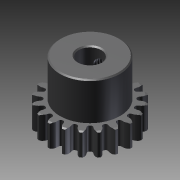
# Autodesk Inventor part: GEAB1.0-20-6-B-6_b
Saved by Autodesk Inventor 2011 SP1 (Build 150282100, 282)
## iProperties
Created: 2016-10-27
Part Number: GEAB1.0-20-6-B-6_b
Catalog Web Link: www.cadenas.de
Description: GEAHB1.0, GEAHBB1.0, GEAHBG1.0, GEAHS1.0, GEAB1.0, GEABB1.0, GEABG1.0, GEAS1.0, GEAKB1.0, GEAKBB1.0, GEAKBG1.0, GEAKS1.0_body-Spur Gears - Pressure Angle 20 Degree Module 1.0
Vendor: MISUMI
Document SubType Name: Modeling
Designer: psAdmin
Manufacturer: MISUMI
Mass: 3.35084 g
Surface Area: 21.074 cm^2
Volume: 3.35084 cm^3
Density: 1 g/cm^3
Category: PARTsolutions
Company: MISUMI
Title: GEAB1.0-20-6-B-6
Author: Cadenas PARTsolutions
Comments: Spur Gears - Pressure Angle 20 Degree Module 1.0
PSOL_IDENT_0: {$CADENAS_DATA\23d-libs\misumi\metric\54_spur_gears\geab10\geab10.prj},460 {VTYP=3D},{NB=GEAB1.0-20-
PSOL_IDENT_1: 6-B-6_b},{LINA=GEAB1.0-20-6-B-6},{NN=GEAHB1.0, GEAHBB1.0, GEAHBG1.0, GEAHS1.0, GEAB1.0, GEABB1.0, GE
PSOL_IDENT_2: ABG1.0, GEAS1.0, GEAKB1.0, GEAKBB1.0, GEAKBG1.0, GEAKS1.0_body},{DATE=13.09.2016 11:19:06},{GEOMDATE=
PSOL_IDENT_3: 13.09.2016 06:08:24},{VERSION=},{LINEID=20},{LINESUBID=-1},{WBVAR=SHS,MAT,ST,NT,B,TS,PS,ALT1,ALT2,TP
PSOL_IDENT_4: C,ALT11,ALT10,BS,ALT4,Z,J,ALT5,Q,R,S,T,ALT9,SRG,ALT6,LFC,LTC,MALT6,ALT7,KFC,KTC,K,ALT3,DIRALT3,QFC,Q
PSOL_IDENT_5: TC,MALT3,ALT8,DIRALT8,ZFC,ZTC,U}  {NB=GEAB1.0-20-6-B-6_b},{LINA=GEAB1.0-20-6-B-6},{KT=DUMMY},{PN=GEA
PSOL_IDENT_6: B1.0-20-6-B-6},{SHS=RHT},{TYPE=GEAB},{MAT=S45C},{MATALG= 'S45C','S45C Equivalent','SUS304','SUS304'
PSOL_IDENT_7: },{ST=},{STALG= '','-','BO','Black Oxide','ENP','Electroless Nickel Plating'},{AC=Set Screw(4137 All
PSOL_IDENT_8: oy Steel Black Oxide)},{MOD=1.0},{NT=20},{NTALG=12,13,14,15,16,17,18,19,20,21,22,23,24,25,26,27,28,2
PSOL_IDENT_9: 9,30,32,34,35,36,38,40,42,44,45,46,48,50,52,54,55,56,58,60,62,64,65,66,68,70,72,75,80,84,85,90,95,96
PSOL_IDENT_10: ,100,110,120},{B=6},{BALG=6,8,10,12},{TS=B},{TSALG='B','B'},{TSPN=-B},{PS=6},{PSALG='6','6','6.35','
PSOL_IDENT_11: 6.35','7','7','8','8','9','9','10','10'},{P=6.00},{DD=20},{D=22},{G=17.5},{H=16},{L=16},{LL1=10},{LL
PSOL_IDENT_12: 2=4},{M=M4},{ML=5.000},{ALT1=},{ALT1ALG='', 'w/o Set Screw', 'KC90','with KC90 (Set Screw)','KC120','
PSOL_IDENT_13: with KC120 (Set Screw)' },{ALT1PN=},{KC=0},{ALT2=},{ALT2ALG= '','w/o TPC (Tapped Hole Dimension)','T
PSOL_IDENT_14: PC','with TPC (Tapped Hole Dimension)' },{TPC=N/A},{TPCALG= 'N/A' },{ALT2PN=},{ALT11=},{ALT11ALG= ''
PSOL_IDENT_15: , 'w/o GBA (Gear bottom adjustment of phase focus)','GBA','with GBA (Gear bottom adjustment of phase
PSOL_IDENT_16: focus)' },{ALT11PN=},{DEG=0},{ALT10=},{ALT10ALG= '','w/o BS (Boss Cut)','BS','with BS (Boss Cut)' }
PSOL_IDENT_17: ,{BS=0.0},{BSALG=0},{BSMIN=7},{BSMAX=10},{ALT10PN=},{LL13D=10},{LL23D=12},{LBS=16},{ALT4=},{ALT4ALG=
PSOL_IDENT_18: '','N/A' },{ALT41=0},{ALT42=0},{ALT4PN=},{Z=0},{ZALG=0},{ZPN=},{ZMINL=8},{ZMAXL=13},{ZMINR=8},{ZMAX
PSOL_IDENT_19: R=12},{J=0.0},{JALG=0},{JPN=},{JMIN=2.0},{JMAX=0.0},{ALT5=},{ALT5ALG= '','N/A' },{ALT5PN=},{Q=0},{QA
PSOL_IDENT_20: LG=0},{QPN=},{QMIN=8},{QMAX=12},{R=0},{RALG=0},{RPN=},{RMIN=8},{RMAX=12.0},{S=0},{SALG=0},{SPN=},{SM
PSOL_IDENT_21: IN=3},{SMAX=10},{T=0},{TALG=0},{TPN=},{TMIN=3},{TMAX=0},{ALT9=},{ALT9ALG= '','Not applicable' },{SRG=
PSOL_IDENT_22: 0.0},{SRGALG=0},{SRGMIN=3.500},{SRGMINALG=3.500},{SRGMAX=0.000},{SRGMAXALG=0.000},{DD2=0.0},{MM=0.00
PSOL_IDENT_23: },{NN=0.00},{DD2ALG=0.000},{MMALG=0.000},{NNALG=0.000},{ALT9PN=},{ALT6=},{ALT6ALG= '','N/A' },{ALT6P
PSOL_IDENT_24: N=},{LFC=0},{LFCALG=0},{LTC=0},{LTCALG=0},{LPCDMIN=14},{LPCDMAX=10},{MALT6=N/A},{MALT6ALG= 'N/A' },{
PSOL_IDENT_25: C=0.0},{ALT7=},{ALT7ALG= '','Not applicable' },{ALT7PN=},{KFC=0},{KFCALG=[0]},{KTC=0},{KTCALG=[0]},{
PSOL_IDENT_26: KPCDMIN1=13},{KPCDMAX1=9},{KPCDMIN2=23},{KPCDMAX2=10},{KPCD=0},{K=0.0},{KALG=[0]},{KALT7L=6},{SCREW=
PSOL_IDENT_27: 4},{SCREWL=5},{ALT3=},{ALT3ALG= '','Not applicable' },{DIRALT3=},{DIRALT3ALG= '','N/A' },{ALT3PN=},{
PSOL_IDENT_28: QFC=0},{QFCALG=[0]},{QTC=0},{QTCALG=[0]},{QPCDMIN1=13},{QPCDMAX1=9},{QPCDMIN2=23},{QPCDMAX2=10},{CIF
PSOL_IDENT_29: MALT3=3},{QPCD=0},{MALT3=N/A},{MALT3ALG= 'N/A' },{MALT3L=0},{MS1=3},{PITCH=0},{BB=0},{TT=0},{ALT8=},
PSOL_IDENT_30: {ALT8ALG= '','Not applicable' },{DIRALT8=},{DIRALT8ALG= '','N/A' },{ALT8PN=},{ZFC=0},{ZFCALG=[0]},{Z
PSOL_IDENT_31: FCMIN=16},{ZFCMAX=7},{ZTC=0},{ZTCALG=[0]},{ZPCDMIN1=16},{ZPCDMIN2=27},{ZPCDMAX1=5},{ZPCDMAX2=7},{ZPC
PSOL_IDENT_32: D=0},{U=0},{UALG=[0]},{UMAX=0},{UMAX1=0},{UMAX2=6},{UMIN=3},{U1=0.0},{U2=0.0},{F=0.0},{PLANE=3},{BL1=
PSOL_IDENT_33: 0},{BL2=15.5},{PCD=0},{SHN=0},{SHDEG1=0},{SHDEG2=0},{PZQRDD2=6},{ALT3LBS=15.5},{D1=4.5},{D2=9},{D3=2
PSOL_IDENT_34: 0},{D4=0.1},{D5=3.333333},{D6=3.076923},{D7=0.85},{D8=0.5},{D9=0.814203},{S1=15},{S2=0.5},{KR=18.16}
NN: 0.00
NT: 20
NB: GEAB1.0-20-6-B-6_b
NBSYN: $PN._b
LINA: GEAB1.0-20-6-B-6
PN: GEAB1.0-20-6-B-6
SHS: Round Hole+Tap
MAT: S45C Equivalent
ST: -
AC: Set Screw(4137 Alloy Steel Black Oxide)
MOD: 1.0
B: 6
TS: B
PS: 6
DD: 20
D: 22
G: 17.5
H: 16
L: 16
LL1: 10
LL2: 4
M: M4
ALT1: w/o Set Screw
ALT2: w/o TPC (Tapped Hole Dimension)
TPC: N/A
ALT11: w/o GBA (Gear bottom adjustment of phase focus)
ALT10: w/o BS (Boss Cut)
BS: 0.0
ALT4: N/A
Z: 0
J: 0.0
ALT5: N/A
Q: 0
R: 0
S: 0
T: 0
ALT9: Not applicable
SRG: 0.0
DD2: 0.0
MM: 0.00
ALT6: N/A
LFC: 0
LTC: 0
MALT6: N/A
C: 0.0
ALT7: Not applicable
KFC: 0
KTC: 0
K: 0.0
ALT3: Not applicable
DIRALT3: N/A
QFC: 0
QTC: 0
MALT3: N/A
ALT8: Not applicable
DIRALT8: N/A
ZFC: 0
ZTC: 0
U: 0
U1: 0.0
U2: 0.0
F: 0.0
SUPPLIER: MISUMI
ARTICLENO: GEAB1.0-20-6-B-6_b
BOMINFO: GEAB1.0-20-6-B-6
CREATOR: CADENAS GmbH
Autodesk Inventor part; units mm, degrees
sketch "Sketch_2" plane through (0, 0, 0) normal (1, 0, 0) x (0, 1, 0)
  line L0 (0, -500) -> (0, 500)
  line L1 (0, 16) -> (7.7, 16)
  line L2 (7.7, 16) -> (8, 15.7)
  line L3 (8, 15.7) -> (8, 6)
  line L4 (8, 6) -> (10.5, 6)
  line L5 (10.5, 6) -> (16, 4.5263)
  line L6 (16, 4.5263) -> (16, 1.4737)
  line L7 (16, 1.4737) -> (10.5, 0)
  line L8 (10.5, 0) -> (0, 0)
  line L9 (0, 0) -> (0, 16)
  constraints: 20 end point
revolve "Revolution1" add sketch "Sketch_2" angle 360 about axis through (0, 0, -500) along (0, 0, -1)
sketch "Sketch_3" plane through (0, 0, 0) normal (0, 0, 1) x (1, 0, 0)
  circle A0 centre (0, 0) radius 44
  arc A1 (-10.9972, 0.248) -> (-10.9972, -0.248) centre (0, 0) ccw
  arc A2 (-10.9972, -0.248) -> (-10.9535, -0.3284) centre (-10.8972, -0.2457) ccw
  arc A3 (-10.9535, -0.3284) -> (-9.9692, -0.7846) centre (-9.0784, 2.4275) ccw
  arc A4 (-9.9692, -0.7846) -> (-9.7201, -0.8136) centre (-9.7516, 0) ccw
  arc A5 (-9.0629, -0.8592) -> (-9.7201, -0.8136) centre (-9.6034, -3.8883) ccw
  arc A6 (-8.6561, -1.2784) -> (-9.0629, -0.8592) centre (-9.1507, -1.3514) ccw
  arc A7 (-8.6561, -1.2784) -> (-8.6275, -1.4591) centre (0, 0) ccw
  arc A8 (-8.8849, -1.9834) -> (-8.6275, -1.4591) centre (-9.1205, -1.5424) ccw
  arc A9 (-9.4958, -2.2299) -> (-8.8849, -1.9834) centre (-10.3349, 0.7304) ccw
  arc A10 (-9.4958, -2.2299) -> (-9.7237, -2.3345) centre (-9.2743, -3.0134) ccw
  arc A11 (-9.7237, -2.3345) -> (-10.5189, -3.0725) centre (-7.8839, -5.1141) ccw
  arc A12 (-10.5189, -3.0725) -> (-10.5356, -3.1625) centre (-10.4398, -3.1337) ccw
  arc A13 (-10.5356, -3.1625) -> (-10.3823, -3.6342) centre (0, 0) ccw
  arc A14 (-10.3823, -3.6342) -> (-10.3159, -3.6971) centre (-10.2879, -3.6011) ccw
  arc A15 (-10.3159, -3.6971) -> (-9.2388, -3.8268) centre (-9.3842, -0.4967) ccw
  arc A16 (-9.2388, -3.8268) -> (-8.993, -3.7775) centre (-9.2743, -3.0134) ccw
  arc A17 (-8.3538, -3.6178) -> (-8.993, -3.7775) centre (-7.9318, -6.6656) ccw
  arc A18 (-7.8374, -3.8907) -> (-8.3538, -3.6178) centre (-8.2853, -4.113) ccw
  arc A19 (-7.8374, -3.8907) -> (-7.7544, -4.0537) centre (0, 0) ccw
  arc A20 (-7.8371, -4.6319) -> (-7.7544, -4.0537) centre (-8.1975, -4.2853) ccw
  arc A21 (-8.342, -5.0551) -> (-7.8371, -4.6319) centre (-10.0548, -2.499) ccw
  arc A22 (-8.342, -5.0551) -> (-8.5264, -5.225) centre (-7.8892, -5.7318) ccw
  arc A23 (-8.5264, -5.225) -> (-9.0546, -6.1726) centre (-5.9177, -7.3) ccw
  arc A24 (-9.0546, -6.1726) -> (-9.0427, -6.2634) centre (-8.9605, -6.2064) ccw
  arc A25 (-9.0427, -6.2634) -> (-8.7512, -6.6646) centre (0, 0) ccw
  arc A26 (-8.7512, -6.6646) -> (-8.6685, -6.704) centre (-8.6716, -6.604) ccw
  arc A27 (-8.6685, -6.704) -> (-7.6041, -6.4945) centre (-8.7714, -3.3722) ccw
  arc A28 (-7.6041, -6.4945) -> (-7.3855, -6.3716) centre (-7.8892, -5.7318) ccw
  arc A29 (-6.827, -6.0222) -> (-7.3855, -6.3716) centre (-5.4838, -8.7904) ccw
  arc A30 (-6.2515, -6.1222) -> (-6.827, -6.0222) centre (-6.6088, -6.472) ccw
  arc A31 (-6.2515, -6.1222) -> (-6.1222, -6.2515) centre (0, 0) ccw
  arc A32 (-6.0222, -6.827) -> (-6.1222, -6.2515) centre (-6.472, -6.6088) ccw
  arc A33 (-6.3716, -7.3855) -> (-6.0222, -6.827) centre (-8.7904, -5.4838) ccw
  arc A34 (-6.3716, -7.3855) -> (-6.4945, -7.6041) centre (-5.7318, -7.8892) ccw
  arc A35 (-6.4945, -7.6041) -> (-6.704, -8.6685) centre (-3.3722, -8.7714) ccw
  arc A36 (-6.704, -8.6685) -> (-6.6646, -8.7512) centre (-6.604, -8.6716) ccw
  arc A37 (-6.6646, -8.7512) -> (-6.2634, -9.0427) centre (0, 0) ccw
  arc A38 (-6.2634, -9.0427) -> (-6.1726, -9.0546) centre (-6.2064, -8.9605) ccw
  arc A39 (-6.1726, -9.0546) -> (-5.225, -8.5264) centre (-7.3, -5.9177) ccw
  arc A40 (-5.225, -8.5264) -> (-5.0551, -8.342) centre (-5.7318, -7.8892) ccw
  arc A41 (-4.6319, -7.8371) -> (-5.0551, -8.342) centre (-2.499, -10.0548) ccw
  arc A42 (-4.0537, -7.7544) -> (-4.6319, -7.8371) centre (-4.2853, -8.1975) ccw
  arc A43 (-4.0537, -7.7544) -> (-3.8907, -7.8374) centre (0, 0) ccw
  arc A44 (-3.6178, -8.3538) -> (-3.8907, -7.8374) centre (-4.113, -8.2853) ccw
  arc A45 (-3.7775, -8.993) -> (-3.6178, -8.3538) centre (-6.6656, -7.9318) ccw
  arc A46 (-3.7775, -8.993) -> (-3.8268, -9.2388) centre (-3.0134, -9.2743) ccw
  arc A47 (-3.8268, -9.2388) -> (-3.6971, -10.3159) centre (-0.4967, -9.3842) ccw
  arc A48 (-3.6971, -10.3159) -> (-3.6342, -10.3823) centre (-3.6011, -10.2879) ccw
  arc A49 (-3.6342, -10.3823) -> (-3.1625, -10.5356) centre (0, 0) ccw
  arc A50 (-3.1625, -10.5356) -> (-3.0725, -10.5189) centre (-3.1337, -10.4398) ccw
  arc A51 (-3.0725, -10.5189) -> (-2.3345, -9.7237) centre (-5.1141, -7.8839) ccw
  arc A52 (-2.3345, -9.7237) -> (-2.2299, -9.4958) centre (-3.0134, -9.2743) ccw
  arc A53 (-1.9834, -8.8849) -> (-2.2299, -9.4958) centre (0.7304, -10.3349) ccw
  arc A54 (-1.4591, -8.6275) -> (-1.9834, -8.8849) centre (-1.5424, -9.1205) ccw
  arc A55 (-1.4591, -8.6275) -> (-1.2784, -8.6561) centre (0, 0) ccw
  arc A56 (-0.8592, -9.0629) -> (-1.2784, -8.6561) centre (-1.3514, -9.1507) ccw
  arc A57 (-0.8136, -9.7201) -> (-0.8592, -9.0629) centre (-3.8883, -9.6034) ccw
  arc A58 (-0.8136, -9.7201) -> (-0.7846, -9.9692) centre (0, -9.7516) ccw
  arc A59 (-0.7846, -9.9692) -> (-0.3284, -10.9535) centre (2.4275, -9.0784) ccw
  arc A60 (-0.3284, -10.9535) -> (-0.248, -10.9972) centre (-0.2457, -10.8972) ccw
  arc A61 (-0.248, -10.9972) -> (0.248, -10.9972) centre (0, 0) ccw
  arc A62 (0.248, -10.9972) -> (0.3284, -10.9535) centre (0.2457, -10.8972) ccw
  arc A63 (0.3284, -10.9535) -> (0.7846, -9.9692) centre (-2.4275, -9.0784) ccw
  arc A64 (0.7846, -9.9692) -> (0.8136, -9.7201) centre (0, -9.7516) ccw
  arc A65 (0.8592, -9.0629) -> (0.8136, -9.7201) centre (3.8883, -9.6034) ccw
  arc A66 (1.2784, -8.6561) -> (0.8592, -9.0629) centre (1.3514, -9.1507) ccw
  arc A67 (1.2784, -8.6561) -> (1.4591, -8.6275) centre (0, 0) ccw
  arc A68 (1.9834, -8.8849) -> (1.4591, -8.6275) centre (1.5424, -9.1205) ccw
  arc A69 (2.2299, -9.4958) -> (1.9834, -8.8849) centre (-0.7304, -10.3349) ccw
  arc A70 (2.2299, -9.4958) -> (2.3345, -9.7237) centre (3.0134, -9.2743) ccw
  arc A71 (2.3345, -9.7237) -> (3.0725, -10.5189) centre (5.1141, -7.8839) ccw
  arc A72 (3.0725, -10.5189) -> (3.1625, -10.5356) centre (3.1337, -10.4398) ccw
  arc A73 (3.1625, -10.5356) -> (3.6342, -10.3823) centre (0, 0) ccw
  arc A74 (3.6342, -10.3823) -> (3.6971, -10.3159) centre (3.6011, -10.2879) ccw
  arc A75 (3.6971, -10.3159) -> (3.8268, -9.2388) centre (0.4967, -9.3842) ccw
  arc A76 (3.8268, -9.2388) -> (3.7775, -8.993) centre (3.0134, -9.2743) ccw
  arc A77 (3.6178, -8.3538) -> (3.7775, -8.993) centre (6.6656, -7.9318) ccw
  arc A78 (3.8907, -7.8374) -> (3.6178, -8.3538) centre (4.113, -8.2853) ccw
  arc A79 (3.8907, -7.8374) -> (4.0537, -7.7544) centre (0, 0) ccw
  arc A80 (4.6319, -7.8371) -> (4.0537, -7.7544) centre (4.2853, -8.1975) ccw
  arc A81 (5.0551, -8.342) -> (4.6319, -7.8371) centre (2.499, -10.0548) ccw
  arc A82 (5.0551, -8.342) -> (5.225, -8.5264) centre (5.7318, -7.8892) ccw
  arc A83 (5.225, -8.5264) -> (6.1726, -9.0546) centre (7.3, -5.9177) ccw
  arc A84 (6.1726, -9.0546) -> (6.2634, -9.0427) centre (6.2064, -8.9605) ccw
  arc A85 (6.2634, -9.0427) -> (6.6646, -8.7512) centre (0, 0) ccw
  arc A86 (6.6646, -8.7512) -> (6.704, -8.6685) centre (6.604, -8.6716) ccw
  arc A87 (6.704, -8.6685) -> (6.4945, -7.6041) centre (3.3722, -8.7714) ccw
  arc A88 (6.4945, -7.6041) -> (6.3716, -7.3855) centre (5.7318, -7.8892) ccw
  arc A89 (6.0222, -6.827) -> (6.3716, -7.3855) centre (8.7904, -5.4838) ccw
  arc A90 (6.1222, -6.2515) -> (6.0222, -6.827) centre (6.472, -6.6088) ccw
  arc A91 (6.1222, -6.2515) -> (6.2515, -6.1222) centre (0, 0) ccw
  arc A92 (6.827, -6.0222) -> (6.2515, -6.1222) centre (6.6088, -6.472) ccw
  arc A93 (7.3855, -6.3716) -> (6.827, -6.0222) centre (5.4838, -8.7904) ccw
  arc A94 (7.3855, -6.3716) -> (7.6041, -6.4945) centre (7.8892, -5.7318) ccw
  arc A95 (7.6041, -6.4945) -> (8.6685, -6.704) centre (8.7714, -3.3722) ccw
  arc A96 (8.6685, -6.704) -> (8.7512, -6.6646) centre (8.6716, -6.604) ccw
  arc A97 (8.7512, -6.6646) -> (9.0427, -6.2634) centre (0, 0) ccw
  arc A98 (9.0427, -6.2634) -> (9.0546, -6.1726) centre (8.9605, -6.2064) ccw
  arc A99 (9.0546, -6.1726) -> (8.5264, -5.225) centre (5.9177, -7.3) ccw
  arc A100 (8.5264, -5.225) -> (8.342, -5.0551) centre (7.8892, -5.7318) ccw
  arc A101 (7.8371, -4.6319) -> (8.342, -5.0551) centre (10.0548, -2.499) ccw
  arc A102 (7.7544, -4.0537) -> (7.8371, -4.6319) centre (8.1975, -4.2853) ccw
  arc A103 (7.7544, -4.0537) -> (7.8374, -3.8907) centre (0, 0) ccw
  arc A104 (8.3538, -3.6178) -> (7.8374, -3.8907) centre (8.2853, -4.113) ccw
  arc A105 (8.993, -3.7775) -> (8.3538, -3.6178) centre (7.9318, -6.6656) ccw
  arc A106 (8.993, -3.7775) -> (9.2388, -3.8268) centre (9.2743, -3.0134) ccw
  arc A107 (9.2388, -3.8268) -> (10.3159, -3.6971) centre (9.3842, -0.4967) ccw
  arc A108 (10.3159, -3.6971) -> (10.3823, -3.6342) centre (10.2879, -3.6011) ccw
  arc A109 (10.3823, -3.6342) -> (10.5356, -3.1625) centre (0, 0) ccw
  arc A110 (10.5356, -3.1625) -> (10.5189, -3.0725) centre (10.4398, -3.1337) ccw
  arc A111 (10.5189, -3.0725) -> (9.7237, -2.3345) centre (7.8839, -5.1141) ccw
  arc A112 (9.7237, -2.3345) -> (9.4958, -2.2299) centre (9.2743, -3.0134) ccw
  arc A113 (8.8849, -1.9834) -> (9.4958, -2.2299) centre (10.3349, 0.7304) ccw
  arc A114 (8.6275, -1.4591) -> (8.8849, -1.9834) centre (9.1205, -1.5424) ccw
  arc A115 (8.6275, -1.4591) -> (8.6561, -1.2784) centre (0, 0) ccw
  arc A116 (9.0629, -0.8592) -> (8.6561, -1.2784) centre (9.1507, -1.3514) ccw
  arc A117 (9.7201, -0.8136) -> (9.0629, -0.8592) centre (9.6034, -3.8883) ccw
  arc A118 (9.7201, -0.8136) -> (9.9692, -0.7846) centre (9.7516, 0) ccw
  arc A119 (9.9692, -0.7846) -> (10.9535, -0.3284) centre (9.0784, 2.4275) ccw
  arc A120 (10.9535, -0.3284) -> (10.9972, -0.248) centre (10.8972, -0.2457) ccw
  arc A121 (10.9972, -0.248) -> (10.9972, 0.248) centre (0, 0) ccw
  arc A122 (10.9972, 0.248) -> (10.9535, 0.3284) centre (10.8972, 0.2457) ccw
  arc A123 (10.9535, 0.3284) -> (9.9692, 0.7846) centre (9.0784, -2.4275) ccw
  arc A124 (9.9692, 0.7846) -> (9.7201, 0.8136) centre (9.7516, 0) ccw
  arc A125 (9.0629, 0.8592) -> (9.7201, 0.8136) centre (9.6034, 3.8883) ccw
  arc A126 (8.6561, 1.2784) -> (9.0629, 0.8592) centre (9.1507, 1.3514) ccw
  arc A127 (8.6561, 1.2784) -> (8.6275, 1.4591) centre (0, 0) ccw
  arc A128 (8.8849, 1.9834) -> (8.6275, 1.4591) centre (9.1205, 1.5424) ccw
  arc A129 (9.4958, 2.2299) -> (8.8849, 1.9834) centre (10.3349, -0.7304) ccw
  arc A130 (9.4958, 2.2299) -> (9.7237, 2.3345) centre (9.2743, 3.0134) ccw
  arc A131 (9.7237, 2.3345) -> (10.5189, 3.0725) centre (7.8839, 5.1141) ccw
  arc A132 (10.5189, 3.0725) -> (10.5356, 3.1625) centre (10.4398, 3.1337) ccw
  arc A133 (10.5356, 3.1625) -> (10.3823, 3.6342) centre (0, 0) ccw
  arc A134 (10.3823, 3.6342) -> (10.3159, 3.6971) centre (10.2879, 3.6011) ccw
  arc A135 (10.3159, 3.6971) -> (9.2388, 3.8268) centre (9.3842, 0.4967) ccw
  arc A136 (9.2388, 3.8268) -> (8.993, 3.7775) centre (9.2743, 3.0134) ccw
  arc A137 (8.3538, 3.6178) -> (8.993, 3.7775) centre (7.9318, 6.6656) ccw
  arc A138 (7.8374, 3.8907) -> (8.3538, 3.6178) centre (8.2853, 4.113) ccw
  arc A139 (7.8374, 3.8907) -> (7.7544, 4.0537) centre (0, 0) ccw
  arc A140 (7.8371, 4.6319) -> (7.7544, 4.0537) centre (8.1975, 4.2853) ccw
  arc A141 (8.342, 5.0551) -> (7.8371, 4.6319) centre (10.0548, 2.499) ccw
  arc A142 (8.342, 5.0551) -> (8.5264, 5.225) centre (7.8892, 5.7318) ccw
  arc A143 (8.5264, 5.225) -> (9.0546, 6.1726) centre (5.9177, 7.3) ccw
  arc A144 (9.0546, 6.1726) -> (9.0427, 6.2634) centre (8.9605, 6.2064) ccw
  arc A145 (9.0427, 6.2634) -> (8.7512, 6.6646) centre (0, 0) ccw
  arc A146 (8.7512, 6.6646) -> (8.6685, 6.704) centre (8.6716, 6.604) ccw
  arc A147 (8.6685, 6.704) -> (7.6041, 6.4945) centre (8.7714, 3.3722) ccw
  arc A148 (7.6041, 6.4945) -> (7.3855, 6.3716) centre (7.8892, 5.7318) ccw
  arc A149 (6.827, 6.0222) -> (7.3855, 6.3716) centre (5.4838, 8.7904) ccw
  arc A150 (6.2515, 6.1222) -> (6.827, 6.0222) centre (6.6088, 6.472) ccw
  arc A151 (6.2515, 6.1222) -> (6.1222, 6.2515) centre (0, 0) ccw
  arc A152 (6.0222, 6.827) -> (6.1222, 6.2515) centre (6.472, 6.6088) ccw
  arc A153 (6.3716, 7.3855) -> (6.0222, 6.827) centre (8.7904, 5.4838) ccw
  arc A154 (6.3716, 7.3855) -> (6.4945, 7.6041) centre (5.7318, 7.8892) ccw
  arc A155 (6.4945, 7.6041) -> (6.704, 8.6685) centre (3.3722, 8.7714) ccw
  arc A156 (6.704, 8.6685) -> (6.6646, 8.7512) centre (6.604, 8.6716) ccw
  arc A157 (6.6646, 8.7512) -> (6.2634, 9.0427) centre (0, 0) ccw
  arc A158 (6.2634, 9.0427) -> (6.1726, 9.0546) centre (6.2064, 8.9605) ccw
  arc A159 (6.1726, 9.0546) -> (5.225, 8.5264) centre (7.3, 5.9177) ccw
  arc A160 (5.225, 8.5264) -> (5.0551, 8.342) centre (5.7318, 7.8892) ccw
  arc A161 (4.6319, 7.8371) -> (5.0551, 8.342) centre (2.499, 10.0548) ccw
  arc A162 (4.0537, 7.7544) -> (4.6319, 7.8371) centre (4.2853, 8.1975) ccw
  arc A163 (4.0537, 7.7544) -> (3.8907, 7.8374) centre (0, 0) ccw
  arc A164 (3.6178, 8.3538) -> (3.8907, 7.8374) centre (4.113, 8.2853) ccw
  arc A165 (3.7775, 8.993) -> (3.6178, 8.3538) centre (6.6656, 7.9318) ccw
  arc A166 (3.7775, 8.993) -> (3.8268, 9.2388) centre (3.0134, 9.2743) ccw
  arc A167 (3.8268, 9.2388) -> (3.6971, 10.3159) centre (0.4967, 9.3842) ccw
  arc A168 (3.6971, 10.3159) -> (3.6342, 10.3823) centre (3.6011, 10.2879) ccw
  arc A169 (3.6342, 10.3823) -> (3.1625, 10.5356) centre (0, 0) ccw
  arc A170 (3.1625, 10.5356) -> (3.0725, 10.5189) centre (3.1337, 10.4398) ccw
  arc A171 (3.0725, 10.5189) -> (2.3345, 9.7237) centre (5.1141, 7.8839) ccw
  arc A172 (2.3345, 9.7237) -> (2.2299, 9.4958) centre (3.0134, 9.2743) ccw
  arc A173 (1.9834, 8.8849) -> (2.2299, 9.4958) centre (-0.7304, 10.3349) ccw
  arc A174 (1.4591, 8.6275) -> (1.9834, 8.8849) centre (1.5424, 9.1205) ccw
  arc A175 (1.4591, 8.6275) -> (1.2784, 8.6561) centre (0, 0) ccw
  arc A176 (0.8592, 9.0629) -> (1.2784, 8.6561) centre (1.3514, 9.1507) ccw
  arc A177 (0.8136, 9.7201) -> (0.8592, 9.0629) centre (3.8883, 9.6034) ccw
  arc A178 (0.8136, 9.7201) -> (0.7846, 9.9692) centre (0, 9.7516) ccw
  arc A179 (0.7846, 9.9692) -> (0.3284, 10.9535) centre (-2.4275, 9.0784) ccw
  arc A180 (0.3284, 10.9535) -> (0.248, 10.9972) centre (0.2457, 10.8972) ccw
  arc A181 (0.248, 10.9972) -> (-0.248, 10.9972) centre (0, 0) ccw
  arc A182 (-0.248, 10.9972) -> (-0.3284, 10.9535) centre (-0.2457, 10.8972) ccw
  arc A183 (-0.3284, 10.9535) -> (-0.7846, 9.9692) centre (2.4275, 9.0784) ccw
  arc A184 (-0.7846, 9.9692) -> (-0.8136, 9.7201) centre (0, 9.7516) ccw
  arc A185 (-0.8592, 9.0629) -> (-0.8136, 9.7201) centre (-3.8883, 9.6034) ccw
  arc A186 (-1.2784, 8.6561) -> (-0.8592, 9.0629) centre (-1.3514, 9.1507) ccw
  arc A187 (-1.2784, 8.6561) -> (-1.4591, 8.6275) centre (0, 0) ccw
  arc A188 (-1.9834, 8.8849) -> (-1.4591, 8.6275) centre (-1.5424, 9.1205) ccw
  arc A189 (-2.2299, 9.4958) -> (-1.9834, 8.8849) centre (0.7304, 10.3349) ccw
  arc A190 (-2.2299, 9.4958) -> (-2.3345, 9.7237) centre (-3.0134, 9.2743) ccw
  arc A191 (-2.3345, 9.7237) -> (-3.0725, 10.5189) centre (-5.1141, 7.8839) ccw
  arc A192 (-3.0725, 10.5189) -> (-3.1625, 10.5356) centre (-3.1337, 10.4398) ccw
  arc A193 (-3.1625, 10.5356) -> (-3.6342, 10.3823) centre (0, 0) ccw
  arc A194 (-3.6342, 10.3823) -> (-3.6971, 10.3159) centre (-3.6011, 10.2879) ccw
  arc A195 (-3.6971, 10.3159) -> (-3.8268, 9.2388) centre (-0.4967, 9.3842) ccw
  arc A196 (-3.8268, 9.2388) -> (-3.7775, 8.993) centre (-3.0134, 9.2743) ccw
  arc A197 (-3.6178, 8.3538) -> (-3.7775, 8.993) centre (-6.6656, 7.9318) ccw
  arc A198 (-3.8907, 7.8374) -> (-3.6178, 8.3538) centre (-4.113, 8.2853) ccw
  arc A199 (-3.8907, 7.8374) -> (-4.0537, 7.7544) centre (0, 0) ccw
  arc A200 (-4.6319, 7.8371) -> (-4.0537, 7.7544) centre (-4.2853, 8.1975) ccw
  arc A201 (-5.0551, 8.342) -> (-4.6319, 7.8371) centre (-2.499, 10.0548) ccw
  arc A202 (-5.0551, 8.342) -> (-5.225, 8.5264) centre (-5.7318, 7.8892) ccw
  arc A203 (-5.225, 8.5264) -> (-6.1726, 9.0546) centre (-7.3, 5.9177) ccw
  arc A204 (-6.1726, 9.0546) -> (-6.2634, 9.0427) centre (-6.2064, 8.9605) ccw
  arc A205 (-6.2634, 9.0427) -> (-6.6646, 8.7512) centre (0, 0) ccw
  arc A206 (-6.6646, 8.7512) -> (-6.704, 8.6685) centre (-6.604, 8.6716) ccw
  arc A207 (-6.704, 8.6685) -> (-6.4945, 7.6041) centre (-3.3722, 8.7714) ccw
  arc A208 (-6.4945, 7.6041) -> (-6.3716, 7.3855) centre (-5.7318, 7.8892) ccw
  arc A209 (-6.0222, 6.827) -> (-6.3716, 7.3855) centre (-8.7904, 5.4838) ccw
  arc A210 (-6.1222, 6.2515) -> (-6.0222, 6.827) centre (-6.472, 6.6088) ccw
  arc A211 (-6.1222, 6.2515) -> (-6.2515, 6.1222) centre (0, 0) ccw
  arc A212 (-6.827, 6.0222) -> (-6.2515, 6.1222) centre (-6.6088, 6.472) ccw
  arc A213 (-7.3855, 6.3716) -> (-6.827, 6.0222) centre (-5.4838, 8.7904) ccw
  arc A214 (-7.3855, 6.3716) -> (-7.6041, 6.4945) centre (-7.8892, 5.7318) ccw
  arc A215 (-7.6041, 6.4945) -> (-8.6685, 6.704) centre (-8.7714, 3.3722) ccw
  arc A216 (-8.6685, 6.704) -> (-8.7512, 6.6646) centre (-8.6716, 6.604) ccw
  arc A217 (-8.7512, 6.6646) -> (-9.0427, 6.2634) centre (0, 0) ccw
  arc A218 (-9.0427, 6.2634) -> (-9.0546, 6.1726) centre (-8.9605, 6.2064) ccw
  arc A219 (-9.0546, 6.1726) -> (-8.5264, 5.225) centre (-5.9177, 7.3) ccw
  arc A220 (-8.5264, 5.225) -> (-8.342, 5.0551) centre (-7.8892, 5.7318) ccw
  arc A221 (-7.8371, 4.6319) -> (-8.342, 5.0551) centre (-10.0548, 2.499) ccw
  arc A222 (-7.7544, 4.0537) -> (-7.8371, 4.6319) centre (-8.1975, 4.2853) ccw
  arc A223 (-7.7544, 4.0537) -> (-7.8374, 3.8907) centre (0, 0) ccw
  arc A224 (-8.3538, 3.6178) -> (-7.8374, 3.8907) centre (-8.2853, 4.113) ccw
  arc A225 (-8.993, 3.7775) -> (-8.3538, 3.6178) centre (-7.9318, 6.6656) ccw
  arc A226 (-8.993, 3.7775) -> (-9.2388, 3.8268) centre (-9.2743, 3.0134) ccw
  arc A227 (-9.2388, 3.8268) -> (-10.3159, 3.6971) centre (-9.3842, 0.4967) ccw
  arc A228 (-10.3159, 3.6971) -> (-10.3823, 3.6342) centre (-10.2879, 3.6011) ccw
  arc A229 (-10.3823, 3.6342) -> (-10.5356, 3.1625) centre (0, 0) ccw
  arc A230 (-10.5356, 3.1625) -> (-10.5189, 3.0725) centre (-10.4398, 3.1337) ccw
  arc A231 (-10.5189, 3.0725) -> (-9.7237, 2.3345) centre (-7.8839, 5.1141) ccw
  arc A232 (-9.7237, 2.3345) -> (-9.4958, 2.2299) centre (-9.2743, 3.0134) ccw
  arc A233 (-8.8849, 1.9834) -> (-9.4958, 2.2299) centre (-10.3349, -0.7304) ccw
  arc A234 (-8.6275, 1.4591) -> (-8.8849, 1.9834) centre (-9.1205, 1.5424) ccw
  arc A235 (-8.6275, 1.4591) -> (-8.6561, 1.2784) centre (0, 0) ccw
  arc A236 (-9.0629, 0.8592) -> (-8.6561, 1.2784) centre (-9.1507, 1.3514) ccw
  arc A237 (-9.7201, 0.8136) -> (-9.0629, 0.8592) centre (-9.6034, 3.8883) ccw
  arc A238 (-9.7201, 0.8136) -> (-9.9692, 0.7846) centre (-9.7516, 0) ccw
  arc A239 (-9.9692, 0.7846) -> (-10.9535, 0.3284) centre (-9.0784, -2.4275) ccw
  arc A240 (-10.9535, 0.3284) -> (-10.9972, 0.248) centre (-10.8972, 0.2457) ccw
  constraints: 480 point on circle, 241 centre point
extrude "Extrusion1" cut sketch "Sketch_3" along normal blind 6
sketch "Sketch3" plane through (0, 0, 0) normal (0, 0, -1) x (-1, 0, 0)
  point P0 (0, 0)
hole "Hole1" at (0, 0, 0) direction (0, 0, 1) diameter 6 depth 16
sketch "_____7" plane through (0, 0, 0) normal (1, 0, 0) x (0, 0, -1)
  line L0 (500, 0) -> (-500, 0)
  line L1 (-0.3, 3) -> (0, 3)
  line L2 (0, 3) -> (0, 3.3)
  line L3 (0, 3.3) -> (-0.3, 3)
  constraints: 8 end point
revolve "Revolution2" cut sketch "_____7" angle 360 about axis through (0, 0, -500) along (0, 0, -1)
sketch "_____17" plane through (0, 0, 0) normal (1, 0, 0) x (0, 0, -1)
  line L0 (500, 0) -> (-500, 0)
  line L1 (-16, 3) -> (-15.7, 3)
  line L2 (-15.7, 3) -> (-16, 3.3)
  line L3 (-16, 3.3) -> (-16, 3)
  constraints: 8 end point
revolve "Revolution3" cut sketch "_____17" angle 360 about axis through (0, 0, -500) along (0, 0, -1)
sketch "Sketch_4" plane through (0, 0, 12) normal (0, 0, 1) x (1, 0, 0)
  line L0 (0, 8) -> (0, 0)
  line L1 (0, 0) -> (-1.621, 0)
  line L2 (-1.621, 0) -> (-1.621, 7.621)
  line L3 (-1.621, 7.621) -> (-2, 8)
  line L4 (-2, 8) -> (0, 8)
  line L5 (0, 8) -> (0, 0)
  constraints: 12 end point
revolve "Revolution4" cut sketch "Sketch_4" angle 360 about axis through (0, 8, 12) along (0, 1, 0)
thread "Thread1" size "M4x0.7" class "6H" standard "ISO Metric profile" length 4.621
ref_plane "b_XY" through (0, 0, 0) normal (0, 0, 1) x (1, 0, 0)
ref_plane "b_YZ" through (0, 0, 0) normal (1, 0, 0) x (0, 1, 0)
ref_plane "b_ZX" through (0, 0, 0) normal (0, 1, 0) x (0, 0, 1)
ref_plane "screw_XY" through (0, 3, 12) normal (0, 1, 0) x (1, 0, 0)
ref_plane "screw_YZ" through (0, 3, 12) normal (1, 0, 0) x (0, 0, -1)
ref_plane "screw_ZX" through (0, 3, 12) normal (0, 0, -1) x (0, 1, 0)
ref_plane "turn_around_XY" through (0, 0, 0) normal (-1, 0, 0) x (0, 0, -1)
ref_plane "turn_around_YZ" through (0, 0, 0) normal (0, 0, -1) x (0, -1, 0)
ref_plane "turn_around_ZX" through (0, 0, 0) normal (0, -1, 0) x (-1, 0, 0)
body "Solid1"
